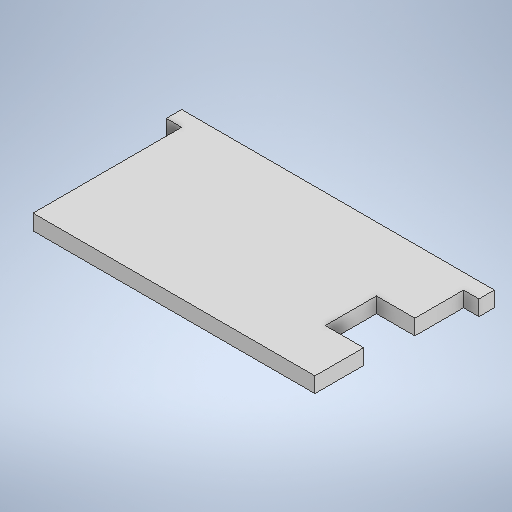
# Autodesk Inventor part: wall 1 for sorting
Saved by Autodesk Inventor 2025.3 (Build 293356000, 356)
## iProperties
Created: 2026-05-24
Part Number: wall 1 for sorting
Material: Generic
Document SubType Name: Modeling
Designer: kamal
Density: 1 g/cm^3
Appearance: Default
Author: kamal
Autodesk Inventor part; units mm, degrees
ref_plane "YZ Plane" through (0, 0, 0) normal (1, 0, 0) x (0, 1, 0)
ref_plane "XZ Plane" through (0, 0, 0) normal (0, 1, 0) x (-1, 0, 0)
ref_plane "XY Plane" through (0, 0, 0) normal (0, 0, 1) x (1, 0, 0)
sketch "Sketch1" plane through (0, 0, 0) normal (0, 1, 0) x (-1, 0, 0)
  line L0 (0, 0) -> (6, 0)
  line L1 (6, 0) -> (6, -6)
  line L2 (6, -6) -> (0, -6)
  line L3 (0, -6) -> (0, 0)
  line L4 (0, -6) -> (-55, -6)
  line L5 (-55, -6) -> (-55, 58)
  line L6 (-55, 58) -> (0, 58)
  line L7 (0, 58) -> (0, -6)
  dimension "d0" = 6
  dimension "d1" = 6
  dimension "d2" = 55
  dimension "d3" = 64
  constraints: 16 end point, 4 parallel, 2 horizontal, 2 perpendicular
  measures "d0" distance of L1.end L2.end
  measures "d1" distance of L0.end L1.end
  measures "d2" distance of L5.end L6.end
  measures "d3" distance of L4.end L5.end
extrude "Extrusion1" add sketch "Sketch1" along normal blind 6
mirror "Mirror1" about plane through (55, 0, 58) normal (1, 0, 0) of "Extrusion1"
sketch "Sketch2" plane through (0, 6, 0) normal (0, 1, 0) x (1, 0, 0)
  line L0 (0, -58) -> (110, -58) projected
  line L1 (0, -58) -> (110, -58) projected
  line L2 (0, -58) -> (110, -58) projected
  line L3 (0, -58) -> (110, -58) projected
  line L4 (-6, 6) -> (-6, 0) projected
  line L5 (-6, 0) -> (0, 0) projected
  line L6 (0, 0) -> (0, -58) projected
  line L7 (0, -58) -> (110, -58) projected
  line L8 (110, 0) -> (110, -58) projected
  line L9 (116, 0) -> (110, 0) projected
  line L10 (116, 6) -> (116, 0) projected
  line L11 (-6, 6) -> (116, 6) projected
  line L12 (-6, 6) -> (116, 6) projected
  line L13 (-6, 6) -> (-6, 0) projected
  line L14 (-6, 6) -> (116, 6) projected
  line L15 (116, 6) -> (116, 0) projected
  line L16 (116, 0) -> (110, 0) projected
  line L17 (110, 0) -> (110, -58) projected
  line L18 (0, -58) -> (110, -58) projected
  line L19 (0, 0) -> (0, -58) projected
  line L20 (-6, 0) -> (0, 0) projected
  line L21 (-6, 6) -> (116, 6) projected
  line L22 (-6, 6) -> (116, 6) projected
  line L23 (-6, 6) -> (116, 6) projected
  line L24 (0, 0) -> (0, -58) projected
  line L25 (0, 0) -> (0, -58) projected
  line L26 (0, 0) -> (0, -58) projected
  line L27 (0, 0) -> (0, -58) projected
  line L28 (-6, 6) -> (-6, 0) projected
  line L29 (-6, 6) -> (-6, 0) projected
  line L30 (-6, 6) -> (-6, 0) projected
  line L31 (-6, 6) -> (-6, 0) projected
  line L32 (-6, 0) -> (0, 0) projected
  line L33 (-6, 0) -> (0, 0) projected
  line L34 (-6, 0) -> (0, 0) projected
  line L35 (-6, 0) -> (0, 0) projected
  line L36 (110, 0) -> (110, -58) projected
  line L37 (110, 0) -> (110, -58) projected
  line L38 (110, 0) -> (110, -58) projected
  line L39 (110, 0) -> (110, -58) projected
  line L40 (116, 0) -> (110, 0) projected
  line L41 (116, 0) -> (110, 0) projected
  line L42 (116, 0) -> (110, 0) projected
  line L43 (116, 0) -> (110, 0) projected
  line L44 (116, 6) -> (116, 0) projected
  line L45 (116, 6) -> (116, 0) projected
  line L46 (116, 6) -> (116, 0) projected
  line L47 (116, 6) -> (116, 0) projected
  line L48 (95, -39) -> (110, -39)
  line L49 (125, -39) -> (125, -19)
  line L50 (125, -19) -> (110, -19)
  line L51 (95, -19) -> (95, -39)
  line L52 (95, -39) -> (125, -19) construction
  line L53 (125, -39) -> (95, -19) construction
  line L54 (110, -19) -> (95, -19)
  line L55 (110, -39) -> (125, -39)
  line L56 (110, -19) -> (110, -39)
  point P0 (110, -29)
  dimension "d6" = 30
  dimension "d7" = 20
  constraints: 18 end point, 5 parallel, 3 midpoint, 3 perpendicular, 2 horizontal, 2 point on line, 2 other
  measures "d6" distance of L51.start L49.end
  measures "d7" distance of L49.end L49.start
extrude "Extrusion2" cut sketch "Sketch2" against normal blind 10 contours L48 L51 L54 L8
body "Solid1"
